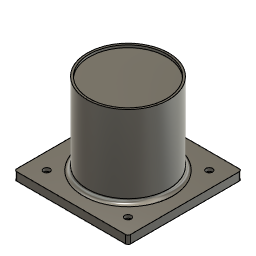
1-base (Autodesk Fusion 360 design; units mm, degrees)
Autodesk Fusion 360 part; units mm, degrees
sketch "Sketch1" plane through (0, 0, 0) normal (0, 1, 0) x (1, 0, 0)
  line L0 (70, -70) -> (-70, -70)
  line L1 (-70, -70) -> (-70, 70)
  line L2 (-70, 70) -> (70, 70)
  line L3 (70, 70) -> (70, -70)
  line L4 (70, -70) -> (-70, 70) construction
  line L5 (-70, -70) -> (70, 70) construction
  dimension "d1" = 140
  dimension "d2" = 140
  constraint horizontal L0
  constraint perpendicular L0 L1
  constraint parallel L0 L2
  constraint parallel L1 L3
  constraint coincident L4 origin
  constraint coincident L5 origin
  measures "d1" distance of L1.end L2.end
  measures "d2" distance of L0.end L1.end
extrude "Extrude1" add sketch "Sketch1" along normal blind 10
sketch "Sketch2" plane through (0, 10, 0) normal (0, 1, 0) x (-1, 0, 0)
  line L0 (-70, -70) -> (70, -70)
  line L1 (70, -70) -> (70, 70)
  line L2 (70, 70) -> (-70, 70)
  line L3 (-70, 70) -> (-70, -70)
  circle A0 centre (0, 0) radius 50
  dimension "d5" = 100
  constraint coincident A0.centre origin
  measures "d5" diameter of A0
extrude "Extrude2" add sketch "Sketch2" along normal blind 100 contours A0
sketch "Sketch3" plane through (0, 0, 0) normal (0, 0, 1) x (1, 0, 0)
  line L0 (-40, 80) -> (40, 80)
  line L1 (40, 80) -> (40, 40)
  line L2 (40, 40) -> (-40, 40)
  line L3 (-40, 40) -> (-40, 80)
  dimension "d8" = 80
  dimension "d9" = 40
  dimension "d10" = 40
  dimension "d11" = 40
  constraint horizontal L0
  constraint vertical L1
  constraint horizontal L2
  constraint vertical L3
  measures "d8" distance of L0.start L0.end
  measures "d9" distance of L0.start L2.end
  measures "d10" horizontal distance of origin L2.end
  measures "d11" distance of origin L2
sketch "Sketch4" plane through (0, 110, 0) normal (0, 1, 0) x (-1, 0, 0)
  circle A0 centre (0, 0) radius 50
  circle A1 centre (0, 0) radius 47.5
  dimension "d14" = 95
  constraint coincident A0.centre A1.centre
  measures "d14" diameter of A1
extrude "Extrude4" cut sketch "Sketch4" against normal blind 3 contours A1
sketch "Sketch5" plane through (0, 10, 0) normal (0, 1, 0) x (-1, 0, 0)
  circle A0 centre (0, 0) radius 50
  line L0 (-70, -70) -> (70, -70)
  line L1 (70, -70) -> (70, 70)
  line L2 (70, 70) -> (-70, 70)
  line L3 (-70, 70) -> (-70, -70)
  point P0 (50, -50)
  point P1 (-50, -50)
  point P2 (-50, 50)
  point P3 (50, 50)
  dimension "d17" = 20
  dimension "d18" = 20
  dimension "d19" = 20
  dimension "d20" = 20
  dimension "d21" = 20
  dimension "d22" = 20
  dimension "d23" = 20
  dimension "d24" = 20
  measures "d17" horizontal distance of L0.end P0
  measures "d18" vertical distance of L0.end P0
  measures "d19" horizontal distance of L0.start P1
  measures "d20" vertical distance of L0.start P1
  measures "d21" horizontal distance of L2.end P2
  measures "d22" vertical distance of L2.end P2
  measures "d23" horizontal distance of L1.end P3
  measures "d24" vertical distance of L1.end P3
hole "Hole1" at (50, 10, -50) at (-50, 10, -50) at (-50, 10, 50) at (50, 10, 50) direction (0, -1, 0) diameter 4.5 depth 40 tip angle 118 counterbore diameter 8 counterbore depth 4
fillet "Fillet1" radius 3 4 edges at (70, 5, 70) (-70, 5, 70) (70, 5, -70) (-70, 5, -70)
fillet "Fillet4" radius 5 1 edges at (46.6164, 10, 18.0808)
